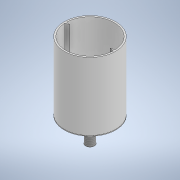
# Autodesk Inventor part: Reactor
Saved by Autodesk Inventor 2022 (Build 260153070, 153G)
## iProperties
Created: 2021-07-20
Part Number: Reactor
Material: Generic
Document SubType Name: Modeling
Designer: Eakawit_kor
Density: 1 g/cm^3
Appearance: Default
Author: Eakawit_kor
Autodesk Inventor part; units mm, degrees
ref_plane "YZ Plane" through (0, 0, 0) normal (1, 0, 0) x (0, 1, 0)
ref_plane "XZ Plane" through (0, 0, 0) normal (0, 1, 0) x (-1, 0, 0)
ref_plane "XY Plane" through (0, 0, 0) normal (0, 0, 1) x (1, 0, 0)
sketch "Sketch1" plane through (0, 0, 0) normal (0, 1, 0) x (-1, 0, 0)
  circle A0 centre (0, 0) radius 25
  circle A1 centre (0, 0) radius 26.6
  line L0 (25, 1) -> (25, 0)
  line L1 (25, 0) -> (25, -1)
  line L2 (25, -1) -> (21, 0)
  line L3 (21, 0) -> (25, 1)
  line L4 (-25, 0) -> (-25, -1)
  line L5 (-25, -1) -> (-21, 0)
  line L6 (-21, 0) -> (-25, 1)
  line L7 (-25, 1) -> (-25, 0)
  point P0 (24.9802, -0.995)
  point P1 (-24.9802, -0.995)
  point P2 (-24.9802, 0.995)
  point P3 (24.9802, 0.995)
  dimension "d0" = 50
  dimension "d1" = 4
  dimension "d2" = 1
  dimension "d3" = 1
  dimension "d4" = 1.6
  dimension "d5" = 1
  dimension "d6" = 1
  dimension "d7" = 4
  constraints: 16 end point, 2 centre point, 2 point on circle, 2 point on line, 2 tangent, 2 vertical, 1 coincident, 1 collinear, 1 equal length
  measures "d0" diameter of A0
  measures "d1" distance from line of L1 L2.end
  measures "d2" distance of L0.end L1.end
  measures "d3" distance of L0.start L0.end
  measures "d4" radial gap between concentric circles of A1 A0
  measures "d5" distance of L4.start L4.end
  measures "d6" distance of L6.end L4.start
  measures "d7" distance of L4.start L5.end
extrude "Extrusion1" add sketch "Sketch1" along normal blind 70 contours A0 L2 L3 | L1 L2 A0 | A0 L3 L0 | L6 L5 A0 | A0 L7 L6 | L5 L4 A0 | A1
sketch "Sketch2" plane through (0, 0, 0) normal (0, 0, 1) x (1, 0, 0)
  line L0 (26.6, 0) -> (-26.6, 0) projected
  line L1 (0.0198, -6.0198) -> (0.0198, -5)
  line L2 (-24.9802, 0) -> (-21, 0) projected
  line L3 (0.0198, -5) -> (-24.9802, 0)
  line L4 (-24.9802, 0) -> (24.9802, 0) projected
  line L5 (-24.9802, 0) -> (-26.6, 0)
  line L6 (-26.6, 0) -> (-26.6, -0.6958)
  line L7 (-26.6, -0.6958) -> (0.0198, -6.0198)
  line L8 (0.0198, -6.0198) -> (0.0198, -26.0198)
  line L9 (0.0198, -26.0198) -> (-4.5302, -26.0198)
  line L10 (-4.5302, -26.0198) -> (-4.5302, -5.1098)
  point P0 (0, 0)
  dimension "d16" = 5
  dimension "d19" = 25
  dimension "d20" = 1
  dimension "d22" = 4.55
  dimension "d23" = 20
  constraints: 16 end point, 3 perpendicular, 2 collinear, 2 point on line, 2 vertical, 1 parallel
  measures "d16" distance from line of L0 L1.end
  measures "d19" distance from line of L2.start L1
  measures "d20" distance between parallel lines of L3 L7
  measures "d22" distance of L8.end L9.end
  measures "d23" distance of L8.start L8.end
revolve "Revolution1" add sketch "Sketch2" angle 360 about axis through (0.0198, -6.0198, 0) along (0, 1, 0)
sketch "Sketch4" plane through (0.0198, -26.0198, 0) normal (0, -1, 0) x (1, 0, 0)
  circle A0 centre (-0.0198, 0) radius 2
  dimension "d24" = 4
  constraints: 1 centre point, 1 coincident
  measures "d24" diameter of A0
extrude "Extrusion3" cut sketch "Sketch4" against normal through all
thread "Thread1" size "M10x1.5" class "6g" standard "ANSI Metric M Profile" length 9
body "Solid1"
